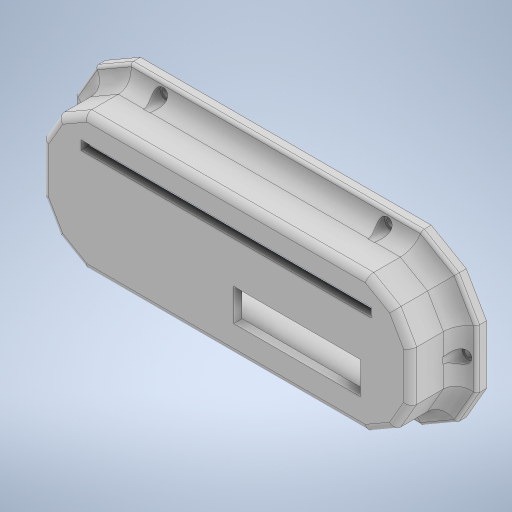
# Autodesk Inventor part: case
Saved by Autodesk Inventor 2024 (Build 280153000, 153)
## iProperties
Created: 2026-05-13
Part Number: case
Material: Generic
Document SubType Name: Modeling
Designer: janst
Density: 1 g/cm^3
Appearance: Default
Author: janst
Autodesk Inventor part; units mm, degrees
ref_plane "YZ Plane" through (0, 0, 0) normal (1, 0, 0) x (0, 1, 0)
ref_plane "XZ Plane" through (0, 0, 0) normal (0, 1, 0) x (-1, 0, 0)
ref_plane "XY Plane" through (0, 0, 0) normal (0, 0, 1) x (1, 0, 0)
sketch "Sketch1" plane through (0, 0, 0) normal (0, 0, 1) x (1, 0, 0)
  line L0 (195.954483, 40.954483) -> (195.954483, 25.954483)
  line L1 (195.954483, 25.954483) -> (186.454483, 9.5)
  line L2 (186.454483, 9.5) -> (170, 0)
  line L3 (170, 0) -> (0, 0)
  line L4 (0, 0) -> (-16.454483, 9.5)
  line L5 (-16.454483, 9.5) -> (-25.954483, 25.954483)
  line L6 (-25.954483, 25.954483) -> (-25.954483, 40.954483)
  line L7 (-25.954483, 40.954483) -> (195.954483, 40.954483)
  line L8 (195.954483, 40.954483) -> (195.954483, 55.954483)
  line L9 (195.954483, 55.954483) -> (186.454483, 72.408965)
  line L10 (186.454483, 72.408965) -> (170, 81.908965)
  line L11 (170, 81.908965) -> (0, 81.908965)
  line L12 (0, 81.908965) -> (-16.454483, 72.408965)
  line L13 (-16.454483, 72.408965) -> (-25.954483, 55.954483)
  line L14 (-25.954483, 55.954483) -> (-25.954483, 40.954483)
  dimension "d5" = 170
  dimension "d7" = 15
  dimension "d9" = 150
  dimension "d11" = 150
  dimension "d13" = 19
  dimension "d14" = 19
  dimension "d16" = 19
  dimension "d17" = 19
  dimension "d18" = 15
  dimension "d19" = 150
  dimension "d20" = 150
  dimension "d21" = 81.90897
  constraints: 30 end point, 7 symmetric about line, 2 coincident, 1 horizontal, 1 parallel, 1 vertical
  measures "d5" distance of L2.end L3.end
  measures "d7" distance of L5.end L6.end
  measures "d9" angle of L3 L2
  measures "d11" angle of L3 L4
  measures "d13" distance of L1.end L2.end
  measures "d14" distance of L3.end L4.end
  measures "d16" distance of L4.end L5.end
  measures "d17" distance of L0.end L1.end
  measures "d18" distance of L0.start L0.end
  measures "d19" angle of L4 L5
  measures "d20" angle of L2 L1
  measures "d21" distance of L3.end L11.end
extrude "Extrusion1" add sketch "Sketch1" along normal blind 5
sketch "Sketch2" plane through (0, 0, 5) normal (0, 0, 1) x (1, 0, 0)
  line L0 (-2.5, 61.408965) -> (172.5, 61.408965)
  line L1 (172.5, 61.408965) -> (172.5, 66.908965)
  line L2 (172.5, 66.908965) -> (-2.5, 66.908965)
  line L3 (-2.5, 66.908965) -> (-2.5, 61.408965)
  line L4 (-2.5, 61.408965) -> (172.5, 66.908965) construction
  line L5 (172.5, 61.408965) -> (-2.5, 66.908965) construction
  line L6 (186.454483, 72.408965) -> (170, 81.908965)
  line L7 (170, 81.908965) -> (0, 81.908965)
  line L8 (0, 81.908965) -> (-16.454483, 72.408965)
  line L9 (-16.454483, 72.408965) -> (-25.954483, 55.954483)
  line L10 (-25.954483, 55.954483) -> (-25.954483, 25.954483)
  line L11 (-25.954483, 25.954483) -> (-16.454483, 9.5)
  line L12 (-16.454483, 9.5) -> (0, 0)
  line L13 (0, 0) -> (170, 0)
  line L14 (170, 0) -> (186.454483, 9.5)
  line L15 (186.454483, 9.5) -> (195.954483, 25.954483)
  line L16 (195.954483, 25.954483) -> (195.954483, 55.954483)
  line L17 (195.954483, 55.954483) -> (186.454483, 72.408965)
  line L18 (85, 94.653689) -> (85, -68.439)
  line L19 (64.545517, 10) -> (4.045517, 10)
  line L20 (4.045517, 10) -> (4.045517, 50)
  line L21 (4.045517, 50) -> (64.545517, 50)
  line L22 (64.545517, 50) -> (64.545517, 10)
  line L23 (64.545517, 10) -> (4.045517, 50) construction
  line L24 (4.045517, 10) -> (64.545517, 50) construction
  line L25 (165.954483, 17) -> (89.554483, 17)
  line L26 (89.554483, 17) -> (89.554483, 36.4)
  line L27 (89.554483, 36.4) -> (165.954483, 36.4)
  line L28 (165.954483, 36.4) -> (165.954483, 17)
  line L29 (165.954483, 17) -> (89.554483, 36.4) construction
  line L30 (89.554483, 17) -> (165.954483, 36.4) construction
  point P0 (85, 64.158965)
  point P1 (34.295517, 30)
  point P2 (127.754483, 26.7)
  dimension "d22" = 175
  dimension "d23" = 5.5
  dimension "d24" = 170
  dimension "d25" = 85
  dimension "d26" = 15
  dimension "d27" = 40
  dimension "d28" = 60.5
  dimension "d29" = 76.4
  dimension "d30" = 19.4
  dimension "d31" = 10
  dimension "d32" = 17
  dimension "d33" = 30
  dimension "d34" = 30
  constraints: 38 end point, 6 midpoint, 6 parallel, 3 horizontal, 3 perpendicular, 1 point on line, 1 vertical
  measures "d22" distance of L1.end L2.end
  measures "d23" distance of L0.end L1.end
  measures "d24" distance of L6.end L7.end
  measures "d25" distance from line of L18 L7.end
  measures "d26" distance between parallel lines of L7 L2
  measures "d27" distance of L21.end L19.start
  measures "d28" distance of L19.start L19.end
  measures "d29" distance of L26.end L27.end
  measures "d30" distance of L25.end L26.end
  measures "d31" distance between parallel lines of L19 L13
  measures "d32" distance between parallel lines of L13 L25
  measures "d33" distance between parallel lines of L16 L28
  measures "d34" distance between parallel lines of L10 L20
extrude "Extrusion2" cut sketch "Sketch2" against normal blind 5 contours L3 L2 L18 L0 | L18 L2 L1 L0
extrude "Extrusion3" cut sketch "Sketch2" against normal blind 5 contours L25 L26 L27 L28
sketch "Sketch3" plane through (0, 0, 0) normal (0, 0, -1) x (-1, 0, 0)
  line L0 (-64.545517, 50) -> (-64.545517, 10)
  line L1 (-4.045517, 50) -> (-64.545517, 50)
  line L2 (-4.045517, 10) -> (-4.045517, 50)
  line L3 (-64.545517, 10) -> (-4.045517, 10)
  point P0 (0, 0)
extrude "Extrusion4" cut sketch "Sketch3" against normal blind 3
sketch "Sketch4" plane through (0, 0, 0) normal (0, 0, -1) x (-1, 0, 0)
  line L0 (0, 0) -> (-170, 0)
  line L1 (16.454483, 9.5) -> (0, 0)
  line L2 (25.954483, 25.954483) -> (16.454483, 9.5)
  line L3 (25.954483, 55.954483) -> (25.954483, 25.954483)
  line L4 (16.454483, 72.408965) -> (25.954483, 55.954483)
  line L5 (0, 81.908965) -> (16.454483, 72.408965)
  line L6 (-170, 81.908965) -> (0, 81.908965)
  line L7 (-186.454483, 72.408965) -> (-170, 81.908965)
  line L8 (-195.954483, 55.954483) -> (-186.454483, 72.408965)
  line L9 (-195.954483, 25.954483) -> (-195.954483, 55.954483)
  line L10 (-186.454483, 9.5) -> (-195.954483, 25.954483)
  line L11 (-170, 0) -> (-186.454483, 9.5)
  line L12 (-0.803848, 78.908965) -> (14.25833, 70.212813)
  line L13 (14.25833, 70.212813) -> (22.954483, 55.150635)
  line L14 (22.954483, 55.150635) -> (22.954483, 26.75833)
  line L15 (22.954483, 26.75833) -> (14.25833, 11.696152)
  line L16 (14.25833, 11.696152) -> (-0.803848, 3)
  line L17 (-0.803848, 3) -> (-169.196152, 3)
  line L18 (-169.196152, 3) -> (-184.25833, 11.696152)
  line L19 (-184.25833, 11.696152) -> (-192.954483, 26.75833)
  line L20 (-192.954483, 26.75833) -> (-192.954483, 55.150635)
  line L21 (-192.954483, 55.150635) -> (-184.25833, 70.212813)
  line L22 (-184.25833, 70.212813) -> (-169.196152, 78.908965)
  line L23 (-169.196152, 78.908965) -> (-0.803848, 78.908965)
  dimension "d41" = 3
  constraints: 24 end point, 11 other
  measures "d41" distance between parallel lines of L6 L23
extrude "Extrusion5" add sketch "Sketch4" along normal blind 25
sketch "Sketch5" plane through (0, 0, -25) normal (0, 0, -1) x (-1, 0, 0)
  line L0 (16.454483, 9.5) -> (25.954483, 25.954483)
  line L1 (25.954483, 25.954483) -> (25.954483, 55.954483)
  line L2 (25.954483, 55.954483) -> (16.454483, 72.408965)
  line L3 (16.454483, 72.408965) -> (0, 81.908965)
  line L4 (0, 81.908965) -> (-170, 81.908965)
  line L5 (-170, 81.908965) -> (-186.454483, 72.408965)
  line L6 (-186.454483, 72.408965) -> (-195.954483, 55.954483)
  line L7 (-195.954483, 55.954483) -> (-195.954483, 25.954483)
  line L8 (-195.954483, 25.954483) -> (-186.454483, 9.5)
  line L9 (-186.454483, 9.5) -> (-170, 0)
  line L10 (-170, 0) -> (0, 0)
  line L11 (0, 0) -> (16.454483, 9.5)
  line L12 (-0.803848, 78.908965) -> (14.25833, 70.212813)
  line L13 (14.25833, 70.212813) -> (22.954483, 55.150635)
  line L14 (22.954483, 55.150635) -> (22.954483, 26.75833)
  line L15 (22.954483, 26.75833) -> (14.25833, 11.696152)
  line L16 (14.25833, 11.696152) -> (-0.803848, 3)
  line L17 (-0.803848, 3) -> (-169.196152, 3)
  line L18 (-169.196152, 3) -> (-184.25833, 11.696152)
  line L19 (-184.25833, 11.696152) -> (-192.954483, 26.75833)
  line L20 (-192.954483, 26.75833) -> (-192.954483, 55.150635)
  line L21 (-192.954483, 55.150635) -> (-184.25833, 70.212813)
  line L22 (-184.25833, 70.212813) -> (-169.196152, 78.908965)
  line L23 (-169.196152, 78.908965) -> (-0.803848, 78.908965)
  line L24 (-172.679492, 91.908965) -> (2.679492, 91.908965)
  line L25 (2.679492, 91.908965) -> (23.774991, 79.729473)
  line L26 (23.774991, 79.729473) -> (35.954483, 58.633975)
  line L27 (35.954483, 58.633975) -> (35.954483, 23.274991)
  line L28 (35.954483, 23.274991) -> (23.774991, 2.179492)
  line L29 (23.774991, 2.179492) -> (2.679492, -10)
  line L30 (2.679492, -10) -> (-172.679492, -10)
  line L31 (-172.679492, -10) -> (-193.774991, 2.179492)
  line L32 (-193.774991, 2.179492) -> (-205.954483, 23.274991)
  line L33 (-205.954483, 23.274991) -> (-205.954483, 58.633975)
  line L34 (-205.954483, 58.633975) -> (-193.774991, 79.729473)
  line L35 (-193.774991, 79.729473) -> (-172.679492, 91.908965)
  dimension "d44" = 10
  constraints: 24 end point, 11 other
  measures "d44" distance between parallel lines of L24 L4
extrude "Extrusion6" add sketch "Sketch5" along normal blind 6 contours L11 L10 L9 L8 L7 L6 L5 L4 L3 L2 L1 L0 | L24 L25 L26 L27 L28 L29 L30 L31 L32 L33 L34 L35
fillet "Fillet1" radius 10 12 edges at (191.2045, 64.1817, -25) (195.9545, 40.9545, -25) (191.2045, 17.7272, -25) (178.2272, 4.75, -25) (85, 0, -25) (-8.2272, 4.75, -25) (-21.2045, 17.7272, -25) (-25.9545, 40.9545, -25) (-21.2045, 64.1817, -25) (-8.2272, 77.159, -25) (85, 81.909, -25) (178.2272, 77.159, -25)
fillet "Fillet2" radius 4 12 edges at (178.2272, 77.159, 5) (85, 81.909, 5) (-8.2272, 77.159, 5) (-21.2045, 64.1817, 5) (-25.9545, 40.9545, 5) (-21.2045, 17.7272, 5) (-8.2272, 4.75, 5) (85, 0, 5) (178.2272, 4.75, 5) (191.2045, 17.7272, 5) (195.9545, 40.9545, 5) (191.2045, 64.1817, 5)
ref_plane "Work Plane1" through (0, 0, -14.75) normal (0, 0, -1) x (-1, 0, 0)
sketch "Sketch6" plane through (0, 0, -14.75) normal (0, 0, -1) x (-1, 0, 0)
  line L0 (-193.774991, 79.729473) -> (-205.954483, 58.633975)
  line L1 (-205.954483, 58.633975) -> (-205.954483, 23.274991)
  line L2 (-205.954483, 23.274991) -> (-193.774991, 2.179492)
  line L3 (-193.774991, 2.179492) -> (-172.679492, -10)
  line L4 (-172.679492, -10) -> (2.679492, -10)
  line L5 (2.679492, -10) -> (23.774991, 2.179492)
  line L6 (23.774991, 2.179492) -> (35.954483, 23.274991)
  line L7 (35.954483, 23.274991) -> (35.954483, 58.633975)
  line L8 (35.954483, 58.633975) -> (23.774991, 79.729473)
  line L9 (23.774991, 79.729473) -> (2.679492, 91.908965)
  line L10 (2.679492, 91.908965) -> (-172.679492, 91.908965)
  line L11 (-172.679492, 91.908965) -> (-193.774991, 79.729473)
  line L12 (-0.803848, 78.908965) -> (14.25833, 70.212813)
  line L13 (14.25833, 70.212813) -> (22.954483, 55.150635)
  line L14 (22.954483, 55.150635) -> (22.954483, 26.75833)
  line L15 (22.954483, 26.75833) -> (14.25833, 11.696152)
  line L16 (14.25833, 11.696152) -> (-0.803848, 3)
  line L17 (-0.803848, 3) -> (-169.196152, 3)
  line L18 (-169.196152, 3) -> (-184.25833, 11.696152)
  line L19 (-184.25833, 11.696152) -> (-192.954483, 26.75833)
  line L20 (-192.954483, 26.75833) -> (-192.954483, 55.150635)
  line L21 (-192.954483, 55.150635) -> (-184.25833, 70.212813)
  line L22 (-184.25833, 70.212813) -> (-169.196152, 78.908965)
  line L23 (-169.196152, 78.908965) -> (-0.803848, 78.908965)
  point P0 (0, 0)
  point P1 (29.864737, 40.954483)
  point P2 (-199.454483, 40.954483)
  point P3 (-17.320508, 85.408965)
  point P4 (-152.679492, 85.408965)
  point P5 (-17.320508, -3.5)
  point P6 (-152.679492, -3.5)
  point P7 (-205.954483, 40.954483)
  dimension "d49" = 13
  dimension "d50" = 6.5
  dimension "d51" = 6.5
  dimension "d52" = 6.5
  dimension "d53" = 6.5
  dimension "d54" = 6.5
  dimension "d55" = 6.08975
  dimension "d56" = 35.35898
  dimension "d57" = 17.67949
  dimension "d58" = 17.67949
  dimension "d59" = 20
  dimension "d60" = 20
  dimension "d61" = 20
  dimension "d62" = 20
  constraints: 1 midpoint
  measures "d49" distance between parallel lines of L17 L4
  measures "d50" distance from line of L4 point (-152.679, -3.5)
  measures "d51" distance from line of L4 point (-17.321, -3.5)
  measures "d52" distance from line of L10 point (-152.679, 85.409)
  measures "d53" distance from line of L10 point (-17.321, 85.409)
  measures "d54" distance of point (-205.954, 40.954) point (-199.454, 40.954)
  measures "d55" distance from line of L7 point (29.865, 40.954)
  measures "d56" distance of L6.end L7.end
  measures "d57" vertical distance of L6.end point (29.865, 40.954)
  measures "d58" vertical distance of L1.end point (-199.454, 40.954)
  measures "d59" horizontal distance of L4.end point (-17.321, -3.5)
  measures "d60" horizontal distance of L3.end point (-152.679, -3.5)
  measures "d61" horizontal distance of point (-17.321, 85.409) L9.end
  measures "d62" horizontal distance of L10.end point (-152.679, 85.409)
hole "Hole1" at (-29.864737, 40.954483, -14.75) at (199.454483, 40.954483, -14.75) at (17.320508, 85.408965, -14.75) at (152.679492, 85.408965, -14.75) at (17.320508, -3.5, -14.75) at (152.679492, -3.5, -14.75) direction (0, 0, -1) diameter 5 end through all counterbore diameter 8 counterbore depth 12
fillet "Fillet3" radius 2 22 edges at (85, 91.9089, -25) (85, 91.909, -25) (-13.2272, 85.8191, -25) (-13.2272, 85.8192, -25) (-29.8647, 69.1817, -25) (-35.9544, 40.9545, -25) (-35.9545, 40.9545, -25) (-29.8647, 12.7273, -25) (-29.8647, 12.7272, -25) (-13.2272, -3.9102, -25) (-13.2272, -3.9103, -25) (85, -9.9999, -25) (85, -10, -25) (183.2272, -3.9102, -25) (183.2272, -3.9103, -25) (199.8647, 12.7273, -25) (199.8647, 12.7272, -25) (205.9544, 40.9545, -25) (205.9545, 40.9545, -25) (199.8647, 69.1817, -25) (183.2272, 85.8191, -25) (183.2272, 85.8192, -25)
chamfer "Chamfer1" distance 2 angle 45 12 edges at (85, 78.909, 0) (176.7272, 74.5609, 0) (188.6064, 62.6817, 0) (192.9545, 40.9545, 0) (188.6064, 19.2272, 0) (176.7272, 7.3481, 0) (85, 3, 0) (-6.7272, 7.3481, 0) (-18.6064, 19.2272, 0) (-22.9545, 40.9545, 0) (-18.6064, 62.6817, 0) (-6.7272, 74.5609, 0)
equation "\"d11\" = d9"
equation "\"d13\" = d14"
equation "\"d16\" = d13"
equation "\"d17\" = d13"
equation "\"d18\" = d7"
equation "\"d19\" = d9"
equation "\"d20\" = d11"
equation "\"d10\" = d8"
equation "\"d8\" = 145deg"
body "Solid1"
